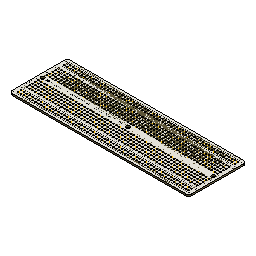
1606 Perma-Proto FullSize (Autodesk Fusion 360 design; units mm, degrees)
Autodesk Fusion 360 part; units mm, degrees
sketch "sketch 305" plane through (0, 0, 0) normal (0, 0, 1) x (1, 0, 0)
  arc A0 (114.3, 22.86) -> (111.76, 25.4) centre (111.76, 22.86) ccw
  line L0 (111.76, 25.4) -> (-40.64, 25.4)
  arc A1 (-40.64, 25.4) -> (-43.18, 22.86) centre (-40.64, 22.86) ccw
  line L1 (-43.18, 22.86) -> (-43.18, -22.86)
  arc A2 (-43.18, -22.86) -> (-40.64, -25.4) centre (-40.64, -22.86) ccw
  line L2 (-40.64, -25.4) -> (111.76, -25.4)
  arc A3 (111.76, -25.4) -> (114.3, -22.86) centre (111.76, -22.86) ccw
  line L3 (114.3, -22.86) -> (114.3, 22.86)
  circle A4 centre (-39.37, 0) radius 1.6
  circle A5 centre (110.49, 0) radius 1.6
  circle A6 centre (35.56, 0) radius 1.6
extrude "Board" add sketch "sketch 305" along normal blind 1.57 makes body 1 in component "Board"
sketch "sketch 5610" plane through (0, 0, 0) normal (0, 0, 1) x (1, 0, 0)
  line L0 (-1.342, -1.4015) -> (1.546, -1.4015)
  line L1 (1.546, -1.4015) -> (1.546, 1.4695)
  line L2 (1.546, 1.4695) -> (-1.342, 1.4695)
  line L3 (-1.342, 1.4695) -> (-1.342, -1.4015)
extrude "ADAFRUIT200MIL" add sketch "sketch 5610" along normal blind 0.1 separate body makes body 2 in component "ADAFRUIT200MIL"
sketch "sketch 5737" plane through (0, 0, 0) normal (0, 0, 1) x (1, 0, 0)
  circle A0 centre (-39.37, -13.97) radius 0.6
  circle A1 centre (-39.37, -11.43) radius 0.6
  circle A2 centre (-39.37, -8.89) radius 0.6
  circle A3 centre (-39.37, -6.35) radius 0.6
  circle A4 centre (-39.37, -3.81) radius 0.6
  circle A5 centre (-36.83, -13.97) radius 0.6
  circle A6 centre (-36.83, -11.43) radius 0.6
  circle A7 centre (-36.83, -8.89) radius 0.6
  circle A8 centre (-36.83, -6.35) radius 0.6
  circle A9 centre (-36.83, -3.81) radius 0.6
  circle A10 centre (-34.29, -13.97) radius 0.6
  circle A11 centre (-34.29, -11.43) radius 0.6
  circle A12 centre (-34.29, -8.89) radius 0.6
  circle A13 centre (-34.29, -6.35) radius 0.6
  circle A14 centre (-34.29, -3.81) radius 0.6
  circle A15 centre (-31.75, -13.97) radius 0.6
  circle A16 centre (-31.75, -11.43) radius 0.6
  circle A17 centre (-31.75, -8.89) radius 0.6
  circle A18 centre (-31.75, -6.35) radius 0.6
  circle A19 centre (-31.75, -3.81) radius 0.6
  circle A20 centre (-29.21, -13.97) radius 0.6
  circle A21 centre (-29.21, -11.43) radius 0.6
  circle A22 centre (-29.21, -8.89) radius 0.6
  circle A23 centre (-29.21, -6.35) radius 0.6
  circle A24 centre (-29.21, -3.81) radius 0.6
  circle A25 centre (-26.67, -13.97) radius 0.6
  circle A26 centre (-26.67, -11.43) radius 0.6
  circle A27 centre (-26.67, -8.89) radius 0.6
  circle A28 centre (-26.67, -6.35) radius 0.6
  circle A29 centre (-26.67, -3.81) radius 0.6
  circle A30 centre (-21.59, -13.97) radius 0.6
  circle A31 centre (-21.59, -11.43) radius 0.6
  circle A32 centre (-21.59, -8.89) radius 0.6
  circle A33 centre (-21.59, -6.35) radius 0.6
  circle A34 centre (-21.59, -3.81) radius 0.6
  circle A35 centre (-24.13, -13.97) radius 0.6
  circle A36 centre (-24.13, -11.43) radius 0.6
  circle A37 centre (-24.13, -8.89) radius 0.6
  circle A38 centre (-24.13, -6.35) radius 0.6
  circle A39 centre (-24.13, -3.81) radius 0.6
  circle A40 centre (-19.05, -13.97) radius 0.6
  circle A41 centre (-19.05, -11.43) radius 0.6
  circle A42 centre (-19.05, -8.89) radius 0.6
  circle A43 centre (-19.05, -6.35) radius 0.6
  circle A44 centre (-19.05, -3.81) radius 0.6
  circle A45 centre (-16.51, -13.97) radius 0.6
  circle A46 centre (-16.51, -11.43) radius 0.6
  circle A47 centre (-16.51, -8.89) radius 0.6
  circle A48 centre (-16.51, -6.35) radius 0.6
  circle A49 centre (-16.51, -3.81) radius 0.6
  circle A50 centre (-13.97, -13.97) radius 0.6
  circle A51 centre (-13.97, -11.43) radius 0.6
  circle A52 centre (-13.97, -8.89) radius 0.6
  circle A53 centre (-13.97, -6.35) radius 0.6
  circle A54 centre (-13.97, -3.81) radius 0.6
  circle A55 centre (-11.43, -13.97) radius 0.6
  circle A56 centre (-11.43, -11.43) radius 0.6
  circle A57 centre (-11.43, -8.89) radius 0.6
  circle A58 centre (-11.43, -6.35) radius 0.6
  circle A59 centre (-11.43, -3.81) radius 0.6
  circle A60 centre (-8.89, -13.97) radius 0.6
  circle A61 centre (-8.89, -11.43) radius 0.6
  circle A62 centre (-8.89, -8.89) radius 0.6
  circle A63 centre (-8.89, -6.35) radius 0.6
  circle A64 centre (-8.89, -3.81) radius 0.6
  circle A65 centre (-6.35, -13.97) radius 0.6
  circle A66 centre (-6.35, -11.43) radius 0.6
  circle A67 centre (-6.35, -8.89) radius 0.6
  circle A68 centre (-6.35, -6.35) radius 0.6
  circle A69 centre (-6.35, -3.81) radius 0.6
  circle A70 centre (-3.81, -13.97) radius 0.6
  circle A71 centre (-3.81, -11.43) radius 0.6
  circle A72 centre (-3.81, -8.89) radius 0.6
  circle A73 centre (-3.81, -6.35) radius 0.6
  circle A74 centre (-3.81, -3.81) radius 0.6
  circle A75 centre (-1.27, -13.97) radius 0.6
  circle A76 centre (-1.27, -11.43) radius 0.6
  circle A77 centre (-1.27, -8.89) radius 0.6
  circle A78 centre (-1.27, -6.35) radius 0.6
  circle A79 centre (-1.27, -3.81) radius 0.6
  circle A80 centre (3.81, -13.97) radius 0.6
  circle A81 centre (3.81, -11.43) radius 0.6
  circle A82 centre (3.81, -8.89) radius 0.6
  circle A83 centre (3.81, -6.35) radius 0.6
  circle A84 centre (3.81, -3.81) radius 0.6
  circle A85 centre (1.27, -13.97) radius 0.6
  circle A86 centre (1.27, -11.43) radius 0.6
  circle A87 centre (1.27, -8.89) radius 0.6
  circle A88 centre (1.27, -6.35) radius 0.6
  circle A89 centre (1.27, -3.81) radius 0.6
  circle A90 centre (6.35, -13.97) radius 0.6
  circle A91 centre (6.35, -11.43) radius 0.6
  circle A92 centre (6.35, -8.89) radius 0.6
  circle A93 centre (6.35, -6.35) radius 0.6
  circle A94 centre (6.35, -3.81) radius 0.6
  circle A95 centre (8.89, -13.97) radius 0.6
  circle A96 centre (8.89, -11.43) radius 0.6
  circle A97 centre (8.89, -8.89) radius 0.6
  circle A98 centre (8.89, -6.35) radius 0.6
  circle A99 centre (8.89, -3.81) radius 0.6
  circle A100 centre (13.97, -13.97) radius 0.6
  circle A101 centre (13.97, -11.43) radius 0.6
  circle A102 centre (13.97, -8.89) radius 0.6
  circle A103 centre (13.97, -6.35) radius 0.6
  circle A104 centre (13.97, -3.81) radius 0.6
  circle A105 centre (11.43, -13.97) radius 0.6
  circle A106 centre (11.43, -11.43) radius 0.6
  circle A107 centre (11.43, -8.89) radius 0.6
  circle A108 centre (11.43, -6.35) radius 0.6
  circle A109 centre (11.43, -3.81) radius 0.6
  circle A110 centre (16.51, -13.97) radius 0.6
  circle A111 centre (16.51, -11.43) radius 0.6
  circle A112 centre (16.51, -8.89) radius 0.6
  circle A113 centre (16.51, -3.81) radius 0.6
  circle A114 centre (16.51, -6.35) radius 0.6
  circle A115 centre (19.05, -13.97) radius 0.6
  circle A116 centre (19.05, -11.43) radius 0.6
  circle A117 centre (19.05, -8.89) radius 0.6
  circle A118 centre (19.05, -6.35) radius 0.6
  circle A119 centre (19.05, -3.81) radius 0.6
  circle A120 centre (21.59, -13.97) radius 0.6
  circle A121 centre (21.59, -11.43) radius 0.6
  circle A122 centre (21.59, -8.89) radius 0.6
  circle A123 centre (21.59, -6.35) radius 0.6
  circle A124 centre (21.59, -3.81) radius 0.6
  circle A125 centre (24.13, -13.97) radius 0.6
  circle A126 centre (24.13, -11.43) radius 0.6
  circle A127 centre (24.13, -8.89) radius 0.6
  circle A128 centre (24.13, -6.35) radius 0.6
  circle A129 centre (24.13, -3.81) radius 0.6
  circle A130 centre (29.21, -13.97) radius 0.6
  circle A131 centre (29.21, -11.43) radius 0.6
  circle A132 centre (29.21, -8.89) radius 0.6
  circle A133 centre (29.21, -6.35) radius 0.6
  circle A134 centre (29.21, -3.81) radius 0.6
  circle A135 centre (26.67, -13.97) radius 0.6
  circle A136 centre (26.67, -11.43) radius 0.6
  circle A137 centre (26.67, -8.89) radius 0.6
  circle A138 centre (26.67, -6.35) radius 0.6
  circle A139 centre (26.67, -3.81) radius 0.6
  circle A140 centre (31.75, -13.97) radius 0.6
  circle A141 centre (31.75, -11.43) radius 0.6
  circle A142 centre (31.75, -8.89) radius 0.6
  circle A143 centre (31.75, -6.35) radius 0.6
  circle A144 centre (31.75, -3.81) radius 0.6
  circle A145 centre (34.29, -13.97) radius 0.6
  circle A146 centre (34.29, -11.43) radius 0.6
  circle A147 centre (34.29, -8.89) radius 0.6
  circle A148 centre (34.29, -6.35) radius 0.6
  circle A149 centre (34.29, -3.81) radius 0.6
  circle A150 centre (-39.37, -19.05) radius 0.6
  circle A151 centre (-36.83, -19.05) radius 0.6
  circle A152 centre (-34.29, -19.05) radius 0.6
  circle A153 centre (-31.75, -19.05) radius 0.6
  circle A154 centre (-29.21, -19.05) radius 0.6
  circle A155 centre (-26.67, -19.05) radius 0.6
  circle A156 centre (-24.13, -19.05) radius 0.6
  circle A157 centre (-21.59, -19.05) radius 0.6
  circle A158 centre (-19.05, -19.05) radius 0.6
  circle A159 centre (-16.51, -19.05) radius 0.6
  circle A160 centre (-13.97, -19.05) radius 0.6
  circle A161 centre (-11.43, -19.05) radius 0.6
  circle A162 centre (-8.89, -19.05) radius 0.6
  circle A163 centre (-6.35, -19.05) radius 0.6
  circle A164 centre (-3.81, -19.05) radius 0.6
  circle A165 centre (-1.27, -19.05) radius 0.6
  circle A166 centre (1.27, -19.05) radius 0.6
  circle A167 centre (3.81, -19.05) radius 0.6
  circle A168 centre (6.35, -19.05) radius 0.6
  circle A169 centre (8.89, -19.05) radius 0.6
  circle A170 centre (11.43, -19.05) radius 0.6
  circle A171 centre (16.51, -19.05) radius 0.6
  circle A172 centre (13.97, -19.05) radius 0.6
  circle A173 centre (19.05, -19.05) radius 0.6
  circle A174 centre (21.59, -19.05) radius 0.6
  circle A175 centre (24.13, -19.05) radius 0.6
  circle A176 centre (26.67, -19.05) radius 0.6
  circle A177 centre (29.21, -19.05) radius 0.6
  circle A178 centre (31.75, -19.05) radius 0.6
  circle A179 centre (34.29, -19.05) radius 0.6
  circle A180 centre (36.83, -19.05) radius 0.6
  circle A181 centre (39.37, -19.05) radius 0.6
  circle A182 centre (41.91, -19.05) radius 0.6
  circle A183 centre (44.45, -19.05) radius 0.6
  circle A184 centre (46.99, -19.05) radius 0.6
  circle A185 centre (49.53, -19.05) radius 0.6
  circle A186 centre (52.07, -19.05) radius 0.6
  circle A187 centre (54.61, -19.05) radius 0.6
  circle A188 centre (57.15, -19.05) radius 0.6
  circle A189 centre (59.69, -19.05) radius 0.6
  circle A190 centre (62.23, -19.05) radius 0.6
  circle A191 centre (64.77, -19.05) radius 0.6
  circle A192 centre (67.31, -19.05) radius 0.6
  circle A193 centre (69.85, -19.05) radius 0.6
  circle A194 centre (72.39, -19.05) radius 0.6
  circle A195 centre (74.93, -19.05) radius 0.6
  circle A196 centre (77.47, -19.05) radius 0.6
  circle A197 centre (80.01, -19.05) radius 0.6
  circle A198 centre (82.55, -19.05) radius 0.6
  circle A199 centre (85.09, -19.05) radius 0.6
  circle A200 centre (87.63, -19.05) radius 0.6
  circle A201 centre (92.71, -19.05) radius 0.6
  circle A202 centre (90.17, -19.05) radius 0.6
  circle A203 centre (95.25, -19.05) radius 0.6
  circle A204 centre (97.79, -19.05) radius 0.6
  circle A205 centre (100.33, -19.05) radius 0.6
  circle A206 centre (102.87, -19.05) radius 0.6
  circle A207 centre (105.41, -19.05) radius 0.6
  circle A208 centre (107.95, -19.05) radius 0.6
  circle A209 centre (110.49, -19.05) radius 0.6
  circle A210 centre (-39.37, -21.59) radius 0.6
  circle A211 centre (-36.83, -21.59) radius 0.6
  circle A212 centre (-34.29, -21.59) radius 0.6
  circle A213 centre (-31.75, -21.59) radius 0.6
  circle A214 centre (-29.21, -21.59) radius 0.6
  circle A215 centre (-26.67, -21.59) radius 0.6
  circle A216 centre (-24.13, -21.59) radius 0.6
  circle A217 centre (-21.59, -21.59) radius 0.6
  circle A218 centre (-19.05, -21.59) radius 0.6
  circle A219 centre (-16.51, -21.59) radius 0.6
  circle A220 centre (-13.97, -21.59) radius 0.6
  circle A221 centre (-11.43, -21.59) radius 0.6
  circle A222 centre (-8.89, -21.59) radius 0.6
  circle A223 centre (-6.35, -21.59) radius 0.6
  circle A224 centre (-3.81, -21.59) radius 0.6
  circle A225 centre (-1.27, -21.59) radius 0.6
  circle A226 centre (1.27, -21.59) radius 0.6
  circle A227 centre (3.81, -21.59) radius 0.6
  circle A228 centre (6.35, -21.59) radius 0.6
  circle A229 centre (8.89, -21.59) radius 0.6
  circle A230 centre (11.43, -21.59) radius 0.6
  circle A231 centre (16.51, -21.59) radius 0.6
  circle A232 centre (13.97, -21.59) radius 0.6
  circle A233 centre (19.05, -21.59) radius 0.6
  circle A234 centre (21.59, -21.59) radius 0.6
  circle A235 centre (24.13, -21.59) radius 0.6
  circle A236 centre (26.67, -21.59) radius 0.6
  circle A237 centre (29.21, -21.59) radius 0.6
  circle A238 centre (31.75, -21.59) radius 0.6
  circle A239 centre (34.29, -21.59) radius 0.6
  circle A240 centre (36.83, -21.59) radius 0.6
  circle A241 centre (39.37, -21.59) radius 0.6
  circle A242 centre (41.91, -21.59) radius 0.6
  circle A243 centre (44.45, -21.59) radius 0.6
  circle A244 centre (46.99, -21.59) radius 0.6
  circle A245 centre (49.53, -21.59) radius 0.6
  circle A246 centre (52.07, -21.59) radius 0.6
  circle A247 centre (54.61, -21.59) radius 0.6
  circle A248 centre (57.15, -21.59) radius 0.6
  circle A249 centre (59.69, -21.59) radius 0.6
  circle A250 centre (62.23, -21.59) radius 0.6
  circle A251 centre (64.77, -21.59) radius 0.6
  circle A252 centre (67.31, -21.59) radius 0.6
  circle A253 centre (69.85, -21.59) radius 0.6
  circle A254 centre (72.39, -21.59) radius 0.6
  circle A255 centre (74.93, -21.59) radius 0.6
  circle A256 centre (77.47, -21.59) radius 0.6
  circle A257 centre (80.01, -21.59) radius 0.6
  circle A258 centre (82.55, -21.59) radius 0.6
  circle A259 centre (85.09, -21.59) radius 0.6
  circle A260 centre (87.63, -21.59) radius 0.6
  circle A261 centre (92.71, -21.59) radius 0.6
  circle A262 centre (90.17, -21.59) radius 0.6
  circle A263 centre (95.25, -21.59) radius 0.6
  circle A264 centre (97.79, -21.59) radius 0.6
  circle A265 centre (100.33, -21.59) radius 0.6
  circle A266 centre (102.87, -21.59) radius 0.6
  circle A267 centre (105.41, -21.59) radius 0.6
  circle A268 centre (107.95, -21.59) radius 0.6
  circle A269 centre (110.49, -21.59) radius 0.6
  circle A270 centre (34.29, 13.97) radius 0.6
  circle A271 centre (34.29, 11.43) radius 0.6
  circle A272 centre (34.29, 8.89) radius 0.6
  circle A273 centre (34.29, 6.35) radius 0.6
  circle A274 centre (34.29, 3.81) radius 0.6
  circle A275 centre (31.75, 13.97) radius 0.6
  circle A276 centre (31.75, 11.43) radius 0.6
  circle A277 centre (31.75, 8.89) radius 0.6
  circle A278 centre (31.75, 6.35) radius 0.6
  circle A279 centre (31.75, 3.81) radius 0.6
  circle A280 centre (29.21, 13.97) radius 0.6
  circle A281 centre (29.21, 11.43) radius 0.6
  circle A282 centre (29.21, 8.89) radius 0.6
  circle A283 centre (29.21, 6.35) radius 0.6
  circle A284 centre (29.21, 3.81) radius 0.6
  circle A285 centre (26.67, 13.97) radius 0.6
  circle A286 centre (26.67, 11.43) radius 0.6
  circle A287 centre (26.67, 8.89) radius 0.6
  circle A288 centre (26.67, 6.35) radius 0.6
  circle A289 centre (26.67, 3.81) radius 0.6
  circle A290 centre (24.13, 13.97) radius 0.6
  circle A291 centre (24.13, 11.43) radius 0.6
  circle A292 centre (24.13, 8.89) radius 0.6
  circle A293 centre (24.13, 6.35) radius 0.6
  circle A294 centre (24.13, 3.81) radius 0.6
  circle A295 centre (21.59, 13.97) radius 0.6
  circle A296 centre (21.59, 11.43) radius 0.6
  circle A297 centre (21.59, 8.89) radius 0.6
  circle A298 centre (21.59, 6.35) radius 0.6
  circle A299 centre (21.59, 3.81) radius 0.6
  circle A300 centre (16.51, 13.97) radius 0.6
  circle A301 centre (16.51, 11.43) radius 0.6
  circle A302 centre (16.51, 8.89) radius 0.6
  circle A303 centre (16.51, 6.35) radius 0.6
  circle A304 centre (16.51, 3.81) radius 0.6
  circle A305 centre (19.05, 13.97) radius 0.6
  circle A306 centre (19.05, 11.43) radius 0.6
  circle A307 centre (19.05, 8.89) radius 0.6
  circle A308 centre (19.05, 6.35) radius 0.6
  circle A309 centre (19.05, 3.81) radius 0.6
  circle A310 centre (13.97, 13.97) radius 0.6
  circle A311 centre (13.97, 11.43) radius 0.6
  circle A312 centre (13.97, 8.89) radius 0.6
  circle A313 centre (13.97, 6.35) radius 0.6
  circle A314 centre (13.97, 3.81) radius 0.6
  circle A315 centre (11.43, 13.97) radius 0.6
  circle A316 centre (11.43, 11.43) radius 0.6
  circle A317 centre (11.43, 8.89) radius 0.6
  circle A318 centre (11.43, 6.35) radius 0.6
  circle A319 centre (11.43, 3.81) radius 0.6
  circle A320 centre (8.89, 13.97) radius 0.6
  circle A321 centre (8.89, 11.43) radius 0.6
  circle A322 centre (8.89, 8.89) radius 0.6
  circle A323 centre (8.89, 6.35) radius 0.6
  circle A324 centre (8.89, 3.81) radius 0.6
  circle A325 centre (6.35, 13.97) radius 0.6
  circle A326 centre (6.35, 11.43) radius 0.6
  circle A327 centre (6.35, 8.89) radius 0.6
  circle A328 centre (6.35, 6.35) radius 0.6
  circle A329 centre (6.35, 3.81) radius 0.6
  circle A330 centre (3.81, 13.97) radius 0.6
  circle A331 centre (3.81, 11.43) radius 0.6
  circle A332 centre (3.81, 8.89) radius 0.6
  circle A333 centre (3.81, 6.35) radius 0.6
  circle A334 centre (3.81, 3.81) radius 0.6
  circle A335 centre (1.27, 13.97) radius 0.6
  circle A336 centre (1.27, 11.43) radius 0.6
  circle A337 centre (1.27, 8.89) radius 0.6
  circle A338 centre (1.27, 6.35) radius 0.6
  circle A339 centre (1.27, 3.81) radius 0.6
  circle A340 centre (-1.27, 13.97) radius 0.6
  circle A341 centre (-1.27, 11.43) radius 0.6
  circle A342 centre (-1.27, 8.89) radius 0.6
  circle A343 centre (-1.27, 6.35) radius 0.6
  circle A344 centre (-1.27, 3.81) radius 0.6
  circle A345 centre (-3.81, 13.97) radius 0.6
  circle A346 centre (-3.81, 11.43) radius 0.6
  circle A347 centre (-3.81, 8.89) radius 0.6
  circle A348 centre (-3.81, 6.35) radius 0.6
  circle A349 centre (-3.81, 3.81) radius 0.6
  circle A350 centre (-8.89, 13.97) radius 0.6
  circle A351 centre (-8.89, 11.43) radius 0.6
  circle A352 centre (-8.89, 8.89) radius 0.6
  circle A353 centre (-8.89, 6.35) radius 0.6
  circle A354 centre (-8.89, 3.81) radius 0.6
  circle A355 centre (-6.35, 13.97) radius 0.6
  circle A356 centre (-6.35, 11.43) radius 0.6
  circle A357 centre (-6.35, 8.89) radius 0.6
  circle A358 centre (-6.35, 6.35) radius 0.6
  circle A359 centre (-6.35, 3.81) radius 0.6
  circle A360 centre (-11.43, 13.97) radius 0.6
  circle A361 centre (-11.43, 11.43) radius 0.6
  circle A362 centre (-11.43, 8.89) radius 0.6
  circle A363 centre (-11.43, 6.35) radius 0.6
  circle A364 centre (-11.43, 3.81) radius 0.6
  circle A365 centre (-13.97, 13.97) radius 0.6
  circle A366 centre (-13.97, 11.43) radius 0.6
  circle A367 centre (-13.97, 8.89) radius 0.6
  circle A368 centre (-13.97, 6.35) radius 0.6
  circle A369 centre (-13.97, 3.81) radius 0.6
  circle A370 centre (-19.05, 13.97) radius 0.6
  circle A371 centre (-19.05, 11.43) radius 0.6
  circle A372 centre (-19.05, 8.89) radius 0.6
  circle A373 centre (-19.05, 6.35) radius 0.6
  circle A374 centre (-19.05, 3.81) radius 0.6
  circle A375 centre (-16.51, 13.97) radius 0.6
  circle A376 centre (-16.51, 11.43) radius 0.6
  circle A377 centre (-16.51, 8.89) radius 0.6
  circle A378 centre (-16.51, 6.35) radius 0.6
  circle A379 centre (-16.51, 3.81) radius 0.6
  circle A380 centre (-21.59, 13.97) radius 0.6
  circle A381 centre (-21.59, 11.43) radius 0.6
  circle A382 centre (-21.59, 8.89) radius 0.6
  circle A383 centre (-21.59, 3.81) radius 0.6
  circle A384 centre (-21.59, 6.35) radius 0.6
  circle A385 centre (-24.13, 13.97) radius 0.6
  circle A386 centre (-24.13, 11.43) radius 0.6
  circle A387 centre (-24.13, 8.89) radius 0.6
  circle A388 centre (-24.13, 6.35) radius 0.6
  circle A389 centre (-24.13, 3.81) radius 0.6
  circle A390 centre (-26.67, 13.97) radius 0.6
  circle A391 centre (-26.67, 11.43) radius 0.6
  circle A392 centre (-26.67, 8.89) radius 0.6
  circle A393 centre (-26.67, 6.35) radius 0.6
  circle A394 centre (-26.67, 3.81) radius 0.6
  circle A395 centre (-29.21, 13.97) radius 0.6
  circle A396 centre (-29.21, 11.43) radius 0.6
  circle A397 centre (-29.21, 8.89) radius 0.6
  circle A398 centre (-29.21, 6.35) radius 0.6
  circle A399 centre (-29.21, 3.81) radius 0.6
  circle A400 centre (-34.29, 13.97) radius 0.6
  circle A401 centre (-34.29, 11.43) radius 0.6
  circle A402 centre (-34.29, 8.89) radius 0.6
  circle A403 centre (-34.29, 6.35) radius 0.6
  circle A404 centre (-34.29, 3.81) radius 0.6
  circle A405 centre (-31.75, 13.97) radius 0.6
  circle A406 centre (-31.75, 11.43) radius 0.6
  circle A407 centre (-31.75, 8.89) radius 0.6
  circle A408 centre (-31.75, 6.35) radius 0.6
  circle A409 centre (-31.75, 3.81) radius 0.6
  circle A410 centre (-36.83, 13.97) radius 0.6
  circle A411 centre (-36.83, 11.43) radius 0.6
  circle A412 centre (-36.83, 8.89) radius 0.6
  circle A413 centre (-36.83, 6.35) radius 0.6
  circle A414 centre (-36.83, 3.81) radius 0.6
  circle A415 centre (-39.37, 13.97) radius 0.6
  circle A416 centre (-39.37, 11.43) radius 0.6
  circle A417 centre (-39.37, 8.89) radius 0.6
  circle A418 centre (-39.37, 6.35) radius 0.6
  circle A419 centre (-39.37, 3.81) radius 0.6
  circle A420 centre (34.29, 19.05) radius 0.6
  circle A421 centre (31.75, 19.05) radius 0.6
  circle A422 centre (29.21, 19.05) radius 0.6
  circle A423 centre (26.67, 19.05) radius 0.6
  circle A424 centre (24.13, 19.05) radius 0.6
  circle A425 centre (21.59, 19.05) radius 0.6
  circle A426 centre (19.05, 19.05) radius 0.6
  circle A427 centre (16.51, 19.05) radius 0.6
  circle A428 centre (13.97, 19.05) radius 0.6
  circle A429 centre (11.43, 19.05) radius 0.6
  circle A430 centre (8.89, 19.05) radius 0.6
  circle A431 centre (6.35, 19.05) radius 0.6
  circle A432 centre (3.81, 19.05) radius 0.6
  circle A433 centre (1.27, 19.05) radius 0.6
  circle A434 centre (-1.27, 19.05) radius 0.6
  circle A435 centre (-3.81, 19.05) radius 0.6
  circle A436 centre (-6.35, 19.05) radius 0.6
  circle A437 centre (-8.89, 19.05) radius 0.6
  circle A438 centre (-11.43, 19.05) radius 0.6
  circle A439 centre (-13.97, 19.05) radius 0.6
  circle A440 centre (-16.51, 19.05) radius 0.6
  circle A441 centre (-21.59, 19.05) radius 0.6
  circle A442 centre (-19.05, 19.05) radius 0.6
  circle A443 centre (-24.13, 19.05) radius 0.6
  circle A444 centre (-26.67, 19.05) radius 0.6
  circle A445 centre (-29.21, 19.05) radius 0.6
  circle A446 centre (-31.75, 19.05) radius 0.6
  circle A447 centre (-34.29, 19.05) radius 0.6
  circle A448 centre (-36.83, 19.05) radius 0.6
  circle A449 centre (-39.37, 19.05) radius 0.6
  circle A450 centre (110.49, 19.05) radius 0.6
  circle A451 centre (107.95, 19.05) radius 0.6
  circle A452 centre (105.41, 19.05) radius 0.6
  circle A453 centre (102.87, 19.05) radius 0.6
  circle A454 centre (100.33, 19.05) radius 0.6
  circle A455 centre (97.79, 19.05) radius 0.6
  circle A456 centre (95.25, 19.05) radius 0.6
  circle A457 centre (92.71, 19.05) radius 0.6
  circle A458 centre (90.17, 19.05) radius 0.6
  circle A459 centre (87.63, 19.05) radius 0.6
  circle A460 centre (85.09, 19.05) radius 0.6
  circle A461 centre (82.55, 19.05) radius 0.6
  circle A462 centre (80.01, 19.05) radius 0.6
  circle A463 centre (77.47, 19.05) radius 0.6
  circle A464 centre (74.93, 19.05) radius 0.6
  circle A465 centre (72.39, 19.05) radius 0.6
  circle A466 centre (69.85, 19.05) radius 0.6
  circle A467 centre (67.31, 19.05) radius 0.6
  circle A468 centre (64.77, 19.05) radius 0.6
  circle A469 centre (62.23, 19.05) radius 0.6
  circle A470 centre (59.69, 19.05) radius 0.6
  circle A471 centre (54.61, 19.05) radius 0.6
  circle A472 centre (57.15, 19.05) radius 0.6
  circle A473 centre (52.07, 19.05) radius 0.6
  circle A474 centre (49.53, 19.05) radius 0.6
  circle A475 centre (46.99, 19.05) radius 0.6
  circle A476 centre (44.45, 19.05) radius 0.6
  circle A477 centre (41.91, 19.05) radius 0.6
  circle A478 centre (39.37, 19.05) radius 0.6
  circle A479 centre (36.83, 19.05) radius 0.6
  circle A480 centre (34.29, 21.59) radius 0.6
  circle A481 centre (31.75, 21.59) radius 0.6
  circle A482 centre (29.21, 21.59) radius 0.6
  circle A483 centre (26.67, 21.59) radius 0.6
  circle A484 centre (24.13, 21.59) radius 0.6
  circle A485 centre (21.59, 21.59) radius 0.6
  circle A486 centre (19.05, 21.59) radius 0.6
  circle A487 centre (16.51, 21.59) radius 0.6
  circle A488 centre (13.97, 21.59) radius 0.6
  circle A489 centre (11.43, 21.59) radius 0.6
  circle A490 centre (8.89, 21.59) radius 0.6
  circle A491 centre (6.35, 21.59) radius 0.6
  circle A492 centre (3.81, 21.59) radius 0.6
  circle A493 centre (1.27, 21.59) radius 0.6
  circle A494 centre (-1.27, 21.59) radius 0.6
  circle A495 centre (-3.81, 21.59) radius 0.6
  circle A496 centre (-6.35, 21.59) radius 0.6
  circle A497 centre (-8.89, 21.59) radius 0.6
  circle A498 centre (-11.43, 21.59) radius 0.6
  circle A499 centre (-13.97, 21.59) radius 0.6
  circle A500 centre (-16.51, 21.59) radius 0.6
  circle A501 centre (-21.59, 21.59) radius 0.6
  circle A502 centre (-19.05, 21.59) radius 0.6
  circle A503 centre (-24.13, 21.59) radius 0.6
  circle A504 centre (-26.67, 21.59) radius 0.6
  circle A505 centre (-29.21, 21.59) radius 0.6
  circle A506 centre (-31.75, 21.59) radius 0.6
  circle A507 centre (-34.29, 21.59) radius 0.6
  circle A508 centre (-36.83, 21.59) radius 0.6
  circle A509 centre (-39.37, 21.59) radius 0.6
  circle A510 centre (110.49, 21.59) radius 0.6
  circle A511 centre (107.95, 21.59) radius 0.6
  circle A512 centre (105.41, 21.59) radius 0.6
  circle A513 centre (102.87, 21.59) radius 0.6
  circle A514 centre (100.33, 21.59) radius 0.6
  circle A515 centre (97.79, 21.59) radius 0.6
  circle A516 centre (95.25, 21.59) radius 0.6
  circle A517 centre (92.71, 21.59) radius 0.6
  circle A518 centre (90.17, 21.59) radius 0.6
  circle A519 centre (87.63, 21.59) radius 0.6
  circle A520 centre (85.09, 21.59) radius 0.6
  circle A521 centre (82.55, 21.59) radius 0.6
  circle A522 centre (80.01, 21.59) radius 0.6
  circle A523 centre (77.47, 21.59) radius 0.6
  circle A524 centre (74.93, 21.59) radius 0.6
  circle A525 centre (72.39, 21.59) radius 0.6
  circle A526 centre (69.85, 21.59) radius 0.6
  circle A527 centre (67.31, 21.59) radius 0.6
  circle A528 centre (64.77, 21.59) radius 0.6
  circle A529 centre (62.23, 21.59) radius 0.6
  circle A530 centre (59.69, 21.59) radius 0.6
  circle A531 centre (54.61, 21.59) radius 0.6
  circle A532 centre (57.15, 21.59) radius 0.6
  circle A533 centre (52.07, 21.59) radius 0.6
  circle A534 centre (49.53, 21.59) radius 0.6
  circle A535 centre (46.99, 21.59) radius 0.6
  circle A536 centre (44.45, 21.59) radius 0.6
  circle A537 centre (41.91, 21.59) radius 0.6
  circle A538 centre (39.37, 21.59) radius 0.6
  circle A539 centre (36.83, 21.59) radius 0.6
  circle A540 centre (36.83, -13.97) radius 0.6
  circle A541 centre (36.83, -11.43) radius 0.6
  circle A542 centre (36.83, -8.89) radius 0.6
  circle A543 centre (36.83, -6.35) radius 0.6
  circle A544 centre (36.83, -3.81) radius 0.6
  circle A545 centre (39.37, -13.97) radius 0.6
  circle A546 centre (39.37, -11.43) radius 0.6
  circle A547 centre (39.37, -8.89) radius 0.6
  circle A548 centre (39.37, -6.35) radius 0.6
  circle A549 centre (39.37, -3.81) radius 0.6
  circle A550 centre (41.91, -13.97) radius 0.6
  circle A551 centre (41.91, -11.43) radius 0.6
  circle A552 centre (41.91, -8.89) radius 0.6
  circle A553 centre (41.91, -6.35) radius 0.6
  circle A554 centre (41.91, -3.81) radius 0.6
  circle A555 centre (44.45, -13.97) radius 0.6
  circle A556 centre (44.45, -11.43) radius 0.6
  circle A557 centre (44.45, -8.89) radius 0.6
  circle A558 centre (44.45, -6.35) radius 0.6
  circle A559 centre (44.45, -3.81) radius 0.6
  circle A560 centre (46.99, -13.97) radius 0.6
  circle A561 centre (46.99, -11.43) radius 0.6
  circle A562 centre (46.99, -8.89) radius 0.6
  circle A563 centre (46.99, -6.35) radius 0.6
  circle A564 centre (46.99, -3.81) radius 0.6
  circle A565 centre (49.53, -13.97) radius 0.6
  circle A566 centre (49.53, -11.43) radius 0.6
  circle A567 centre (49.53, -8.89) radius 0.6
  circle A568 centre (49.53, -6.35) radius 0.6
  circle A569 centre (49.53, -3.81) radius 0.6
  circle A570 centre (54.61, -13.97) radius 0.6
  circle A571 centre (54.61, -11.43) radius 0.6
  circle A572 centre (54.61, -8.89) radius 0.6
  circle A573 centre (54.61, -6.35) radius 0.6
  circle A574 centre (54.61, -3.81) radius 0.6
  circle A575 centre (52.07, -13.97) radius 0.6
  circle A576 centre (52.07, -11.43) radius 0.6
  circle A577 centre (52.07, -8.89) radius 0.6
  circle A578 centre (52.07, -6.35) radius 0.6
  circle A579 centre (52.07, -3.81) radius 0.6
  circle A580 centre (57.15, -13.97) radius 0.6
  circle A581 centre (57.15, -11.43) radius 0.6
  circle A582 centre (57.15, -8.89) radius 0.6
  circle A583 centre (57.15, -6.35) radius 0.6
  circle A584 centre (57.15, -3.81) radius 0.6
  circle A585 centre (59.69, -13.97) radius 0.6
  circle A586 centre (59.69, -11.43) radius 0.6
  circle A587 centre (59.69, -8.89) radius 0.6
  circle A588 centre (59.69, -6.35) radius 0.6
  circle A589 centre (59.69, -3.81) radius 0.6
  circle A590 centre (62.23, -13.97) radius 0.6
  circle A591 centre (62.23, -11.43) radius 0.6
  circle A592 centre (62.23, -8.89) radius 0.6
  circle A593 centre (62.23, -6.35) radius 0.6
  circle A594 centre (62.23, -3.81) radius 0.6
  circle A595 centre (64.77, -13.97) radius 0.6
  circle A596 centre (64.77, -11.43) radius 0.6
  circle A597 centre (64.77, -8.89) radius 0.6
  circle A598 centre (64.77, -6.35) radius 0.6
  circle A599 centre (64.77, -3.81) radius 0.6
  circle A600 centre (67.31, -13.97) radius 0.6
  circle A601 centre (67.31, -11.43) radius 0.6
  circle A602 centre (67.31, -8.89) radius 0.6
  circle A603 centre (67.31, -6.35) radius 0.6
  circle A604 centre (67.31, -3.81) radius 0.6
  circle A605 centre (69.85, -13.97) radius 0.6
  circle A606 centre (69.85, -11.43) radius 0.6
  circle A607 centre (69.85, -8.89) radius 0.6
  circle A608 centre (69.85, -6.35) radius 0.6
  circle A609 centre (69.85, -3.81) radius 0.6
  circle A610 centre (72.39, -13.97) radius 0.6
  circle A611 centre (72.39, -11.43) radius 0.6
  circle A612 centre (72.39, -8.89) radius 0.6
  circle A613 centre (72.39, -6.35) radius 0.6
  circle A614 centre (72.39, -3.81) radius 0.6
  circle A615 centre (74.93, -13.97) radius 0.6
  circle A616 centre (74.93, -11.43) radius 0.6
  circle A617 centre (74.93, -8.89) radius 0.6
  circle A618 centre (74.93, -6.35) radius 0.6
  circle A619 centre (74.93, -3.81) radius 0.6
  circle A620 centre (80.01, -13.97) radius 0.6
  circle A621 centre (80.01, -11.43) radius 0.6
  circle A622 centre (80.01, -8.89) radius 0.6
  circle A623 centre (80.01, -6.35) radius 0.6
  circle A624 centre (80.01, -3.81) radius 0.6
  circle A625 centre (77.47, -13.97) radius 0.6
  circle A626 centre (77.47, -11.43) radius 0.6
  circle A627 centre (77.47, -8.89) radius 0.6
  circle A628 centre (77.47, -6.35) radius 0.6
  circle A629 centre (77.47, -3.81) radius 0.6
  circle A630 centre (82.55, -13.97) radius 0.6
  circle A631 centre (82.55, -11.43) radius 0.6
  circle A632 centre (82.55, -8.89) radius 0.6
  circle A633 centre (82.55, -6.35) radius 0.6
  circle A634 centre (82.55, -3.81) radius 0.6
  circle A635 centre (85.09, -13.97) radius 0.6
  circle A636 centre (85.09, -11.43) radius 0.6
  circle A637 centre (85.09, -8.89) radius 0.6
  circle A638 centre (85.09, -6.35) radius 0.6
  circle A639 centre (85.09, -3.81) radius 0.6
  circle A640 centre (90.17, -13.97) radius 0.6
  circle A641 centre (90.17, -11.43) radius 0.6
  circle A642 centre (90.17, -8.89) radius 0.6
  circle A643 centre (90.17, -6.35) radius 0.6
  circle A644 centre (90.17, -3.81) radius 0.6
  circle A645 centre (87.63, -13.97) radius 0.6
  circle A646 centre (87.63, -11.43) radius 0.6
  circle A647 centre (87.63, -8.89) radius 0.6
  circle A648 centre (87.63, -6.35) radius 0.6
  circle A649 centre (87.63, -3.81) radius 0.6
  circle A650 centre (92.71, -13.97) radius 0.6
  circle A651 centre (92.71, -11.43) radius 0.6
  circle A652 centre (92.71, -8.89) radius 0.6
  circle A653 centre (92.71, -3.81) radius 0.6
  circle A654 centre (92.71, -6.35) radius 0.6
  circle A655 centre (95.25, -13.97) radius 0.6
  circle A656 centre (95.25, -11.43) radius 0.6
  circle A657 centre (95.25, -8.89) radius 0.6
  circle A658 centre (95.25, -6.35) radius 0.6
  circle A659 centre (95.25, -3.81) radius 0.6
  circle A660 centre (97.79, -13.97) radius 0.6
  circle A661 centre (97.79, -11.43) radius 0.6
  circle A662 centre (97.79, -8.89) radius 0.6
  circle A663 centre (97.79, -6.35) radius 0.6
  circle A664 centre (97.79, -3.81) radius 0.6
  circle A665 centre (100.33, -13.97) radius 0.6
  circle A666 centre (100.33, -11.43) radius 0.6
  circle A667 centre (100.33, -8.89) radius 0.6
  circle A668 centre (100.33, -6.35) radius 0.6
  circle A669 centre (100.33, -3.81) radius 0.6
  circle A670 centre (105.41, -13.97) radius 0.6
  circle A671 centre (105.41, -11.43) radius 0.6
  circle A672 centre (105.41, -8.89) radius 0.6
  circle A673 centre (105.41, -6.35) radius 0.6
  circle A674 centre (105.41, -3.81) radius 0.6
  circle A675 centre (102.87, -13.97) radius 0.6
  circle A676 centre (102.87, -11.43) radius 0.6
  circle A677 centre (102.87, -8.89) radius 0.6
  circle A678 centre (102.87, -6.35) radius 0.6
  circle A679 centre (102.87, -3.81) radius 0.6
  circle A680 centre (107.95, -13.97) radius 0.6
  circle A681 centre (107.95, -11.43) radius 0.6
  circle A682 centre (107.95, -8.89) radius 0.6
  circle A683 centre (107.95, -6.35) radius 0.6
  circle A684 centre (107.95, -3.81) radius 0.6
  circle A685 centre (110.49, -13.97) radius 0.6
  circle A686 centre (110.49, -11.43) radius 0.6
  circle A687 centre (110.49, -8.89) radius 0.6
  circle A688 centre (110.49, -6.35) radius 0.6
  circle A689 centre (110.49, -3.81) radius 0.6
  circle A690 centre (110.49, 13.97) radius 0.6
  circle A691 centre (110.49, 11.43) radius 0.6
  circle A692 centre (110.49, 8.89) radius 0.6
  circle A693 centre (110.49, 6.35) radius 0.6
  circle A694 centre (110.49, 3.81) radius 0.6
  circle A695 centre (107.95, 13.97) radius 0.6
  circle A696 centre (107.95, 11.43) radius 0.6
  circle A697 centre (107.95, 8.89) radius 0.6
  circle A698 centre (107.95, 6.35) radius 0.6
  circle A699 centre (107.95, 3.81) radius 0.6
  circle A700 centre (105.41, 13.97) radius 0.6
  circle A701 centre (105.41, 11.43) radius 0.6
  circle A702 centre (105.41, 8.89) radius 0.6
  circle A703 centre (105.41, 6.35) radius 0.6
  circle A704 centre (105.41, 3.81) radius 0.6
  circle A705 centre (102.87, 13.97) radius 0.6
  circle A706 centre (102.87, 11.43) radius 0.6
  circle A707 centre (102.87, 8.89) radius 0.6
  circle A708 centre (102.87, 6.35) radius 0.6
  circle A709 centre (102.87, 3.81) radius 0.6
  circle A710 centre (100.33, 13.97) radius 0.6
  circle A711 centre (100.33, 11.43) radius 0.6
  circle A712 centre (100.33, 8.89) radius 0.6
  circle A713 centre (100.33, 6.35) radius 0.6
  circle A714 centre (100.33, 3.81) radius 0.6
  circle A715 centre (97.79, 13.97) radius 0.6
  circle A716 centre (97.79, 11.43) radius 0.6
  circle A717 centre (97.79, 8.89) radius 0.6
  circle A718 centre (97.79, 6.35) radius 0.6
  circle A719 centre (97.79, 3.81) radius 0.6
  circle A720 centre (92.71, 13.97) radius 0.6
  circle A721 centre (92.71, 11.43) radius 0.6
  circle A722 centre (92.71, 8.89) radius 0.6
  circle A723 centre (92.71, 6.35) radius 0.6
  circle A724 centre (92.71, 3.81) radius 0.6
  circle A725 centre (95.25, 13.97) radius 0.6
  circle A726 centre (95.25, 11.43) radius 0.6
  circle A727 centre (95.25, 8.89) radius 0.6
  circle A728 centre (95.25, 6.35) radius 0.6
  circle A729 centre (95.25, 3.81) radius 0.6
  circle A730 centre (90.17, 13.97) radius 0.6
  circle A731 centre (90.17, 11.43) radius 0.6
  circle A732 centre (90.17, 8.89) radius 0.6
  circle A733 centre (90.17, 6.35) radius 0.6
  circle A734 centre (90.17, 3.81) radius 0.6
  circle A735 centre (87.63, 13.97) radius 0.6
  circle A736 centre (87.63, 11.43) radius 0.6
  circle A737 centre (87.63, 8.89) radius 0.6
  circle A738 centre (87.63, 6.35) radius 0.6
  circle A739 centre (87.63, 3.81) radius 0.6
  circle A740 centre (85.09, 13.97) radius 0.6
  circle A741 centre (85.09, 11.43) radius 0.6
  circle A742 centre (85.09, 8.89) radius 0.6
  circle A743 centre (85.09, 6.35) radius 0.6
  circle A744 centre (85.09, 3.81) radius 0.6
  circle A745 centre (82.55, 13.97) radius 0.6
  circle A746 centre (82.55, 11.43) radius 0.6
  circle A747 centre (82.55, 8.89) radius 0.6
  circle A748 centre (82.55, 6.35) radius 0.6
  circle A749 centre (82.55, 3.81) radius 0.6
  circle A750 centre (80.01, 13.97) radius 0.6
  circle A751 centre (80.01, 11.43) radius 0.6
  circle A752 centre (80.01, 8.89) radius 0.6
  circle A753 centre (80.01, 6.35) radius 0.6
  circle A754 centre (80.01, 3.81) radius 0.6
  circle A755 centre (77.47, 13.97) radius 0.6
  circle A756 centre (77.47, 11.43) radius 0.6
  circle A757 centre (77.47, 8.89) radius 0.6
  circle A758 centre (77.47, 6.35) radius 0.6
  circle A759 centre (77.47, 3.81) radius 0.6
  circle A760 centre (74.93, 13.97) radius 0.6
  circle A761 centre (74.93, 11.43) radius 0.6
  circle A762 centre (74.93, 8.89) radius 0.6
  circle A763 centre (74.93, 6.35) radius 0.6
  circle A764 centre (74.93, 3.81) radius 0.6
  circle A765 centre (72.39, 13.97) radius 0.6
  circle A766 centre (72.39, 11.43) radius 0.6
  circle A767 centre (72.39, 8.89) radius 0.6
  circle A768 centre (72.39, 6.35) radius 0.6
  circle A769 centre (72.39, 3.81) radius 0.6
  circle A770 centre (67.31, 13.97) radius 0.6
  circle A771 centre (67.31, 11.43) radius 0.6
  circle A772 centre (67.31, 8.89) radius 0.6
  circle A773 centre (67.31, 6.35) radius 0.6
  circle A774 centre (67.31, 3.81) radius 0.6
  circle A775 centre (69.85, 13.97) radius 0.6
  circle A776 centre (69.85, 11.43) radius 0.6
  circle A777 centre (69.85, 8.89) radius 0.6
  circle A778 centre (69.85, 6.35) radius 0.6
  circle A779 centre (69.85, 3.81) radius 0.6
  circle A780 centre (64.77, 13.97) radius 0.6
  circle A781 centre (64.77, 11.43) radius 0.6
  circle A782 centre (64.77, 8.89) radius 0.6
  circle A783 centre (64.77, 6.35) radius 0.6
  circle A784 centre (64.77, 3.81) radius 0.6
  circle A785 centre (62.23, 13.97) radius 0.6
  circle A786 centre (62.23, 11.43) radius 0.6
  circle A787 centre (62.23, 8.89) radius 0.6
  circle A788 centre (62.23, 6.35) radius 0.6
  circle A789 centre (62.23, 3.81) radius 0.6
  circle A790 centre (57.15, 13.97) radius 0.6
  circle A791 centre (57.15, 11.43) radius 0.6
  circle A792 centre (57.15, 8.89) radius 0.6
  circle A793 centre (57.15, 6.35) radius 0.6
  circle A794 centre (57.15, 3.81) radius 0.6
  circle A795 centre (59.69, 13.97) radius 0.6
  circle A796 centre (59.69, 11.43) radius 0.6
  circle A797 centre (59.69, 8.89) radius 0.6
  circle A798 centre (59.69, 6.35) radius 0.6
  circle A799 centre (59.69, 3.81) radius 0.6
  circle A800 centre (54.61, 13.97) radius 0.6
  circle A801 centre (54.61, 11.43) radius 0.6
  circle A802 centre (54.61, 8.89) radius 0.6
  circle A803 centre (54.61, 3.81) radius 0.6
  circle A804 centre (54.61, 6.35) radius 0.6
  circle A805 centre (52.07, 13.97) radius 0.6
  circle A806 centre (52.07, 11.43) radius 0.6
  circle A807 centre (52.07, 8.89) radius 0.6
  circle A808 centre (52.07, 6.35) radius 0.6
  circle A809 centre (52.07, 3.81) radius 0.6
  circle A810 centre (49.53, 13.97) radius 0.6
  circle A811 centre (49.53, 11.43) radius 0.6
  circle A812 centre (49.53, 8.89) radius 0.6
  circle A813 centre (49.53, 6.35) radius 0.6
  circle A814 centre (49.53, 3.81) radius 0.6
  circle A815 centre (46.99, 13.97) radius 0.6
  circle A816 centre (46.99, 11.43) radius 0.6
  circle A817 centre (46.99, 8.89) radius 0.6
  circle A818 centre (46.99, 6.35) radius 0.6
  circle A819 centre (46.99, 3.81) radius 0.6
  circle A820 centre (41.91, 13.97) radius 0.6
  circle A821 centre (41.91, 11.43) radius 0.6
  circle A822 centre (41.91, 8.89) radius 0.6
  circle A823 centre (41.91, 6.35) radius 0.6
  circle A824 centre (41.91, 3.81) radius 0.6
  circle A825 centre (44.45, 13.97) radius 0.6
  circle A826 centre (44.45, 11.43) radius 0.6
  circle A827 centre (44.45, 8.89) radius 0.6
  circle A828 centre (44.45, 6.35) radius 0.6
  circle A829 centre (44.45, 3.81) radius 0.6
  circle A830 centre (39.37, 13.97) radius 0.6
  circle A831 centre (39.37, 11.43) radius 0.6
  circle A832 centre (39.37, 8.89) radius 0.6
  circle A833 centre (39.37, 6.35) radius 0.6
  circle A834 centre (39.37, 3.81) radius 0.6
  circle A835 centre (36.83, 13.97) radius 0.6
  circle A836 centre (36.83, 11.43) radius 0.6
  circle A837 centre (36.83, 8.89) radius 0.6
  circle A838 centre (36.83, 6.35) radius 0.6
  circle A839 centre (36.83, 3.81) radius 0.6
extrude "Extrude3" cut sketch "sketch 5737" along normal blind 1.57 bodies 1 in component "Board"
component "PCB Component" placed x (1, 0, 0) y (0, 1, 0) z (0, 0, 1) at (0, 0, 0)
component "Board" placed x (1, 0, 0) y (0, 1, 0) z (0, 0, 1) at (0, 0, 0) in component "PCB Component"
component "ADAFRUIT200MIL" placed x (0, -1, 0) y (1, 0, 0) z (0, 0, 1) at (-34.798, 0.254, 1.57) in component "PCB Component"
named bodies: "Board", "ADAFRUIT200MIL"
